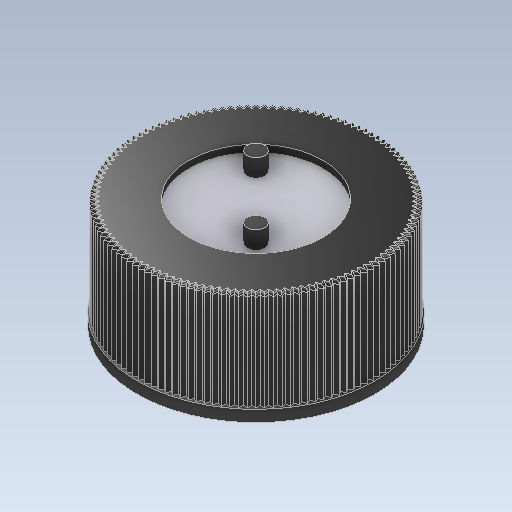
# Autodesk Inventor part: 40ml Bottle 1 lid
Saved by Autodesk Inventor 2021 (Build 250183000, 183)
## iProperties
Created: 2019-11-05
Part Number: 40ml Bottle 1 lid
Material: Generic
Document SubType Name: Modeling
Designer: jgray
Density: 1 g/cm^3
Appearance: Default
Author: jgray
Autodesk Inventor part; units mm, degrees
ref_plane "YZ Plane" through (0, 0, 0) normal (1, 0, 0) x (0, 1, 0)
ref_plane "XZ Plane" through (0, 0, 0) normal (0, 1, 0) x (-1, 0, 0)
ref_plane "XY Plane" through (0, 0, 0) normal (0, 0, 1) x (1, 0, 0)
sketch "Sketch1" plane through (0, 0, 0) normal (0, 1, 0) x (-1, 0, 0)
  circle A0 centre (0, 0) radius 13.35
  dimension "d0" = 26.7
  constraints: 1 centre point, 1 coincident
  measures "d0" diameter of A0
extrude "Extrusion1" add sketch "Sketch1" along normal blind 1.3
sketch "Sketch2" plane through (0, 1.3, 0) normal (0, 1, 0) x (1, 0, 0)
  circle A0 centre (0, 0) radius 13.2
  circle A1 centre (0, 0) radius 12.8 construction
  line L0 (-13.2, 0) -> (-13.1819, 0.6908) construction
  line L1 (-13.1819, 0.6908) -> (-13.1277, 1.3798) construction
  line L2 (-13.1277, 1.3798) -> (-13.0375, 2.0649) construction
  line L3 (-13.0375, 2.0649) -> (-12.9115, 2.7444) construction
  line L4 (-12.9115, 2.7444) -> (-12.7502, 3.4164) construction
  line L5 (-12.7502, 3.4164) -> (-12.5539, 4.079) construction
  line L6 (-12.5539, 4.079) -> (-12.3233, 4.7305) construction
  line L7 (-12.3233, 4.7305) -> (-12.0588, 5.3689) construction
  line L8 (-12.0588, 5.3689) -> (-11.7613, 5.9927) construction
  line L9 (-11.7613, 5.9927) -> (-11.4315, 6.6) construction
  line L10 (-11.4315, 6.6) -> (-11.0705, 7.1892) construction
  line L11 (-11.0705, 7.1892) -> (-10.679, 7.7588) construction
  line L12 (-10.679, 7.7588) -> (-10.2583, 8.307) construction
  line L13 (-10.2583, 8.307) -> (-9.8095, 8.8325) construction
  line L14 (-9.8095, 8.8325) -> (-9.3338, 9.3338) construction
  line L15 (-9.3338, 9.3338) -> (-8.8325, 9.8095) construction
  line L16 (-8.8325, 9.8095) -> (-8.307, 10.2583) construction
  line L17 (-8.307, 10.2583) -> (-7.7588, 10.679) construction
  line L18 (-7.7588, 10.679) -> (-7.1892, 11.0705) construction
  line L19 (-7.1892, 11.0705) -> (-6.6, 11.4315) construction
  line L20 (-6.6, 11.4315) -> (-5.9927, 11.7613) construction
  line L21 (-5.9927, 11.7613) -> (-5.3689, 12.0588) construction
  line L22 (-5.3689, 12.0588) -> (-4.7305, 12.3233) construction
  line L23 (-4.7305, 12.3233) -> (-4.079, 12.5539) construction
  line L24 (-4.079, 12.5539) -> (-3.4164, 12.7502) construction
  line L25 (-3.4164, 12.7502) -> (-2.7444, 12.9115) construction
  line L26 (-2.7444, 12.9115) -> (-2.0649, 13.0375) construction
  line L27 (-2.0649, 13.0375) -> (-1.3798, 13.1277) construction
  line L28 (-1.3798, 13.1277) -> (-0.6908, 13.1819) construction
  line L29 (-0.6908, 13.1819) -> (0, 13.2) construction
  line L30 (0, 13.2) -> (0.6908, 13.1819) construction
  line L31 (0.6908, 13.1819) -> (1.3798, 13.1277) construction
  line L32 (1.3798, 13.1277) -> (2.0649, 13.0375) construction
  line L33 (2.0649, 13.0375) -> (2.7444, 12.9115) construction
  line L34 (2.7444, 12.9115) -> (3.4164, 12.7502) construction
  line L35 (3.4164, 12.7502) -> (4.079, 12.5539) construction
  line L36 (4.079, 12.5539) -> (4.7305, 12.3233) construction
  line L37 (4.7305, 12.3233) -> (5.3689, 12.0588) construction
  line L38 (5.3689, 12.0588) -> (5.9927, 11.7613) construction
  line L39 (5.9927, 11.7613) -> (6.6, 11.4315) construction
  line L40 (6.6, 11.4315) -> (7.1892, 11.0705) construction
  line L41 (7.1892, 11.0705) -> (7.7588, 10.679) construction
  line L42 (7.7588, 10.679) -> (8.307, 10.2583) construction
  line L43 (8.307, 10.2583) -> (8.8325, 9.8095) construction
  line L44 (8.8325, 9.8095) -> (9.3338, 9.3338) construction
  line L45 (9.3338, 9.3338) -> (9.8095, 8.8325) construction
  line L46 (9.8095, 8.8325) -> (10.2583, 8.307) construction
  line L47 (10.2583, 8.307) -> (10.679, 7.7588) construction
  line L48 (10.679, 7.7588) -> (11.0705, 7.1892) construction
  line L49 (11.0705, 7.1892) -> (11.4315, 6.6) construction
  line L50 (11.4315, 6.6) -> (11.7613, 5.9927) construction
  line L51 (11.7613, 5.9927) -> (12.0588, 5.3689) construction
  line L52 (12.0588, 5.3689) -> (12.3233, 4.7305) construction
  line L53 (12.3233, 4.7305) -> (12.5539, 4.079) construction
  line L54 (12.5539, 4.079) -> (12.7502, 3.4164) construction
  line L55 (12.7502, 3.4164) -> (12.9115, 2.7444) construction
  line L56 (12.9115, 2.7444) -> (13.0375, 2.0649) construction
  line L57 (13.0375, 2.0649) -> (13.1277, 1.3798) construction
  line L58 (13.1277, 1.3798) -> (13.1819, 0.6908) construction
  line L59 (13.1819, 0.6908) -> (13.2, 0) construction
  line L60 (13.2, 0) -> (13.1819, -0.6908) construction
  line L61 (13.1819, -0.6908) -> (13.1277, -1.3798) construction
  line L62 (13.1277, -1.3798) -> (13.0375, -2.0649) construction
  line L63 (13.0375, -2.0649) -> (12.9115, -2.7444) construction
  line L64 (12.9115, -2.7444) -> (12.7502, -3.4164) construction
  line L65 (12.7502, -3.4164) -> (12.5539, -4.079) construction
  line L66 (12.5539, -4.079) -> (12.3233, -4.7305) construction
  line L67 (12.3233, -4.7305) -> (12.0588, -5.3689) construction
  line L68 (12.0588, -5.3689) -> (11.7613, -5.9927) construction
  line L69 (11.7613, -5.9927) -> (11.4315, -6.6) construction
  line L70 (11.4315, -6.6) -> (11.0705, -7.1892) construction
  line L71 (11.0705, -7.1892) -> (10.679, -7.7588) construction
  line L72 (10.679, -7.7588) -> (10.2583, -8.307) construction
  line L73 (10.2583, -8.307) -> (9.8095, -8.8325) construction
  line L74 (9.8095, -8.8325) -> (9.3338, -9.3338) construction
  line L75 (9.3338, -9.3338) -> (8.8325, -9.8095) construction
  line L76 (8.8325, -9.8095) -> (8.307, -10.2583) construction
  line L77 (8.307, -10.2583) -> (7.7588, -10.679) construction
  line L78 (7.7588, -10.679) -> (7.1892, -11.0705) construction
  line L79 (7.1892, -11.0705) -> (6.6, -11.4315) construction
  line L80 (6.6, -11.4315) -> (5.9927, -11.7613) construction
  line L81 (5.9927, -11.7613) -> (5.3689, -12.0588) construction
  line L82 (5.3689, -12.0588) -> (4.7305, -12.3233) construction
  line L83 (4.7305, -12.3233) -> (4.079, -12.5539) construction
  line L84 (4.079, -12.5539) -> (3.4164, -12.7502) construction
  line L85 (3.4164, -12.7502) -> (2.7444, -12.9115) construction
  line L86 (2.7444, -12.9115) -> (2.0649, -13.0375) construction
  line L87 (2.0649, -13.0375) -> (1.3798, -13.1277) construction
  line L88 (1.3798, -13.1277) -> (0.6908, -13.1819) construction
  line L89 (0.6908, -13.1819) -> (0, -13.2) construction
  line L90 (0, -13.2) -> (-0.6908, -13.1819) construction
  line L91 (-0.6908, -13.1819) -> (-1.3798, -13.1277) construction
  line L92 (-1.3798, -13.1277) -> (-2.0649, -13.0375) construction
  line L93 (-2.0649, -13.0375) -> (-2.7444, -12.9115) construction
  line L94 (-2.7444, -12.9115) -> (-3.4164, -12.7502) construction
  line L95 (-3.4164, -12.7502) -> (-4.079, -12.5539) construction
  line L96 (-4.079, -12.5539) -> (-4.7305, -12.3233) construction
  line L97 (-4.7305, -12.3233) -> (-5.3689, -12.0588) construction
  line L98 (-5.3689, -12.0588) -> (-5.9927, -11.7613) construction
  line L99 (-5.9927, -11.7613) -> (-6.6, -11.4315) construction
  line L100 (-6.6, -11.4315) -> (-7.1892, -11.0705) construction
  line L101 (-7.1892, -11.0705) -> (-7.7588, -10.679) construction
  line L102 (-7.7588, -10.679) -> (-8.307, -10.2583) construction
  line L103 (-8.307, -10.2583) -> (-8.8325, -9.8095) construction
  line L104 (-8.8325, -9.8095) -> (-9.3338, -9.3338) construction
  line L105 (-9.3338, -9.3338) -> (-9.8095, -8.8325) construction
  line L106 (-9.8095, -8.8325) -> (-10.2583, -8.307) construction
  line L107 (-10.2583, -8.307) -> (-10.679, -7.7588) construction
  line L108 (-10.679, -7.7588) -> (-11.0705, -7.1892) construction
  line L109 (-11.0705, -7.1892) -> (-11.4315, -6.6) construction
  line L110 (-11.4315, -6.6) -> (-11.7613, -5.9927) construction
  line L111 (-11.7613, -5.9927) -> (-12.0588, -5.3689) construction
  line L112 (-12.0588, -5.3689) -> (-12.3233, -4.7305) construction
  line L113 (-12.3233, -4.7305) -> (-12.5539, -4.079) construction
  line L114 (-12.5539, -4.079) -> (-12.7502, -3.4164) construction
  line L115 (-12.7502, -3.4164) -> (-12.9115, -2.7444) construction
  line L116 (-12.9115, -2.7444) -> (-13.0375, -2.0649) construction
  line L117 (-13.0375, -2.0649) -> (-13.1277, -1.3798) construction
  line L118 (-13.1277, -1.3798) -> (-13.1819, -0.6908) construction
  line L119 (-13.1819, -0.6908) -> (-13.2, 0) construction
  line L120 (0, 0) -> (-13.191, -0.3454) construction
  line L121 (-12.7956, -0.3351) -> (-12.7956, 0.3351) construction
  line L122 (-12.7956, 0.3351) -> (-12.7605, 1.0043) construction
  line L123 (-12.7605, 1.0043) -> (-12.6905, 1.6707) construction
  line L124 (-12.6905, 1.6707) -> (-12.5857, 2.3326) construction
  line L125 (-12.5857, 2.3326) -> (-12.4463, 2.9881) construction
  line L126 (-12.4463, 2.9881) -> (-12.2729, 3.6354) construction
  line L127 (-12.2729, 3.6354) -> (-12.0658, 4.2727) construction
  line L128 (-12.0658, 4.2727) -> (-11.8257, 4.8983) construction
  line L129 (-11.8257, 4.8983) -> (-11.5531, 5.5105) construction
  line L130 (-11.5531, 5.5105) -> (-11.2489, 6.1076) construction
  line L131 (-11.2489, 6.1076) -> (-10.9138, 6.688) construction
  line L132 (-10.9138, 6.688) -> (-10.5488, 7.25) construction
  line L133 (-10.5488, 7.25) -> (-10.1549, 7.7921) construction
  line L134 (-10.1549, 7.7921) -> (-9.7332, 8.3129) construction
  line L135 (-9.7332, 8.3129) -> (-9.2848, 8.8109) construction
  line L136 (-9.2848, 8.8109) -> (-8.8109, 9.2848) construction
  line L137 (-8.8109, 9.2848) -> (-8.3129, 9.7332) construction
  line L138 (-8.3129, 9.7332) -> (-7.7921, 10.1549) construction
  line L139 (-7.7921, 10.1549) -> (-7.25, 10.5488) construction
  line L140 (-7.25, 10.5488) -> (-6.688, 10.9138) construction
  line L141 (-6.688, 10.9138) -> (-6.1076, 11.2489) construction
  line L142 (-6.1076, 11.2489) -> (-5.5105, 11.5531) construction
  line L143 (-5.5105, 11.5531) -> (-4.8983, 11.8257) construction
  line L144 (-4.8983, 11.8257) -> (-4.2727, 12.0658) construction
  line L145 (-4.2727, 12.0658) -> (-3.6354, 12.2729) construction
  line L146 (-3.6354, 12.2729) -> (-2.9881, 12.4463) construction
  line L147 (-2.9881, 12.4463) -> (-2.3326, 12.5857) construction
  line L148 (-2.3326, 12.5857) -> (-1.6707, 12.6905) construction
  line L149 (-1.6707, 12.6905) -> (-1.0043, 12.7605) construction
  line L150 (-1.0043, 12.7605) -> (-0.3351, 12.7956) construction
  line L151 (-0.3351, 12.7956) -> (0.3351, 12.7956) construction
  line L152 (0.3351, 12.7956) -> (1.0043, 12.7605) construction
  line L153 (1.0043, 12.7605) -> (1.6707, 12.6905) construction
  line L154 (1.6707, 12.6905) -> (2.3326, 12.5857) construction
  line L155 (2.3326, 12.5857) -> (2.9881, 12.4463) construction
  line L156 (2.9881, 12.4463) -> (3.6354, 12.2729) construction
  line L157 (3.6354, 12.2729) -> (4.2727, 12.0658) construction
  line L158 (4.2727, 12.0658) -> (4.8983, 11.8257) construction
  line L159 (4.8983, 11.8257) -> (5.5105, 11.5531) construction
  line L160 (5.5105, 11.5531) -> (6.1076, 11.2489) construction
  line L161 (6.1076, 11.2489) -> (6.688, 10.9138) construction
  line L162 (6.688, 10.9138) -> (7.25, 10.5488) construction
  line L163 (7.25, 10.5488) -> (7.7921, 10.1549) construction
  line L164 (7.7921, 10.1549) -> (8.3129, 9.7332) construction
  line L165 (8.3129, 9.7332) -> (8.8109, 9.2848) construction
  line L166 (8.8109, 9.2848) -> (9.2848, 8.8109) construction
  line L167 (9.2848, 8.8109) -> (9.7332, 8.3129) construction
  line L168 (9.7332, 8.3129) -> (10.1549, 7.7921) construction
  line L169 (10.1549, 7.7921) -> (10.5488, 7.25) construction
  line L170 (10.5488, 7.25) -> (10.9138, 6.688) construction
  line L171 (10.9138, 6.688) -> (11.2489, 6.1076) construction
  line L172 (11.2489, 6.1076) -> (11.5531, 5.5105) construction
  line L173 (11.5531, 5.5105) -> (11.8257, 4.8983) construction
  line L174 (11.8257, 4.8983) -> (12.0658, 4.2727) construction
  line L175 (12.0658, 4.2727) -> (12.2729, 3.6354) construction
  line L176 (12.2729, 3.6354) -> (12.4463, 2.9881) construction
  line L177 (12.4463, 2.9881) -> (12.5857, 2.3326) construction
  line L178 (12.5857, 2.3326) -> (12.6905, 1.6707) construction
  line L179 (12.6905, 1.6707) -> (12.7605, 1.0043) construction
  line L180 (12.7605, 1.0043) -> (12.7956, 0.3351) construction
  line L181 (12.7956, 0.3351) -> (12.7956, -0.3351) construction
  line L182 (12.7956, -0.3351) -> (12.7605, -1.0043) construction
  line L183 (12.7605, -1.0043) -> (12.6905, -1.6707) construction
  line L184 (12.6905, -1.6707) -> (12.5857, -2.3326) construction
  line L185 (12.5857, -2.3326) -> (12.4463, -2.9881) construction
  line L186 (12.4463, -2.9881) -> (12.2729, -3.6354) construction
  line L187 (12.2729, -3.6354) -> (12.0658, -4.2727) construction
  line L188 (12.0658, -4.2727) -> (11.8257, -4.8983) construction
  line L189 (11.8257, -4.8983) -> (11.5531, -5.5105) construction
  line L190 (11.5531, -5.5105) -> (11.2489, -6.1076) construction
  line L191 (11.2489, -6.1076) -> (10.9138, -6.688) construction
  line L192 (10.9138, -6.688) -> (10.5488, -7.25) construction
  line L193 (10.5488, -7.25) -> (10.1549, -7.7921) construction
  line L194 (10.1549, -7.7921) -> (9.7332, -8.3129) construction
  line L195 (9.7332, -8.3129) -> (9.2848, -8.8109) construction
  line L196 (9.2848, -8.8109) -> (8.8109, -9.2848) construction
  line L197 (8.8109, -9.2848) -> (8.3129, -9.7332) construction
  line L198 (8.3129, -9.7332) -> (7.7921, -10.1549) construction
  line L199 (7.7921, -10.1549) -> (7.25, -10.5488) construction
  line L200 (7.25, -10.5488) -> (6.688, -10.9138) construction
  line L201 (6.688, -10.9138) -> (6.1076, -11.2489) construction
  line L202 (6.1076, -11.2489) -> (5.5105, -11.5531) construction
  line L203 (5.5105, -11.5531) -> (4.8983, -11.8257) construction
  line L204 (4.8983, -11.8257) -> (4.2727, -12.0658) construction
  line L205 (4.2727, -12.0658) -> (3.6354, -12.2729) construction
  line L206 (3.6354, -12.2729) -> (2.9881, -12.4463) construction
  line L207 (2.9881, -12.4463) -> (2.3326, -12.5857) construction
  line L208 (2.3326, -12.5857) -> (1.6707, -12.6905) construction
  line L209 (1.6707, -12.6905) -> (1.0043, -12.7605) construction
  line L210 (1.0043, -12.7605) -> (0.3351, -12.7956) construction
  line L211 (0.3351, -12.7956) -> (-0.3351, -12.7956) construction
  line L212 (-0.3351, -12.7956) -> (-1.0043, -12.7605) construction
  line L213 (-1.0043, -12.7605) -> (-1.6707, -12.6905) construction
  line L214 (-1.6707, -12.6905) -> (-2.3326, -12.5857) construction
  line L215 (-2.3326, -12.5857) -> (-2.9881, -12.4463) construction
  line L216 (-2.9881, -12.4463) -> (-3.6354, -12.2729) construction
  line L217 (-3.6354, -12.2729) -> (-4.2727, -12.0658) construction
  line L218 (-4.2727, -12.0658) -> (-4.8983, -11.8257) construction
  line L219 (-4.8983, -11.8257) -> (-5.5105, -11.5531) construction
  line L220 (-5.5105, -11.5531) -> (-6.1076, -11.2489) construction
  line L221 (-6.1076, -11.2489) -> (-6.688, -10.9138) construction
  line L222 (-6.688, -10.9138) -> (-7.25, -10.5488) construction
  line L223 (-7.25, -10.5488) -> (-7.7921, -10.1549) construction
  line L224 (-7.7921, -10.1549) -> (-8.3129, -9.7332) construction
  line L225 (-8.3129, -9.7332) -> (-8.8109, -9.2848) construction
  line L226 (-8.8109, -9.2848) -> (-9.2848, -8.8109) construction
  line L227 (-9.2848, -8.8109) -> (-9.7332, -8.3129) construction
  line L228 (-9.7332, -8.3129) -> (-10.1549, -7.7921) construction
  line L229 (-10.1549, -7.7921) -> (-10.5488, -7.25) construction
  line L230 (-10.5488, -7.25) -> (-10.9138, -6.688) construction
  line L231 (-10.9138, -6.688) -> (-11.2489, -6.1076) construction
  line L232 (-11.2489, -6.1076) -> (-11.5531, -5.5105) construction
  line L233 (-11.5531, -5.5105) -> (-11.8257, -4.8983) construction
  line L234 (-11.8257, -4.8983) -> (-12.0658, -4.2727) construction
  line L235 (-12.0658, -4.2727) -> (-12.2729, -3.6354) construction
  line L236 (-12.2729, -3.6354) -> (-12.4463, -2.9881) construction
  line L237 (-12.4463, -2.9881) -> (-12.5857, -2.3326) construction
  line L238 (-12.5857, -2.3326) -> (-12.6905, -1.6707) construction
  line L239 (-12.6905, -1.6707) -> (-12.7605, -1.0043) construction
  line L240 (-12.7605, -1.0043) -> (-12.7956, -0.3351) construction
  line L241 (-12.7956, -0.3351) -> (-13.2, 0)
  line L242 (-12.7956, 0.3351) -> (-13.2, 0)
  line L243 (-12.7605, -1.0043) -> (-13.1819, -0.6908)
  line L244 (-12.7956, -0.3351) -> (-13.1819, -0.6908)
  line L245 (-12.6905, -1.6707) -> (-13.1277, -1.3798)
  line L246 (-12.7605, -1.0043) -> (-13.1277, -1.3798)
  line L247 (-12.5857, -2.3326) -> (-13.0375, -2.0649)
  line L248 (-12.6905, -1.6707) -> (-13.0375, -2.0649)
  line L249 (-12.4463, -2.9881) -> (-12.9115, -2.7444)
  line L250 (-12.5857, -2.3326) -> (-12.9115, -2.7444)
  line L251 (-12.2729, -3.6354) -> (-12.7502, -3.4164)
  line L252 (-12.4463, -2.9881) -> (-12.7502, -3.4164)
  line L253 (-12.0658, -4.2727) -> (-12.5539, -4.079)
  line L254 (-12.2729, -3.6354) -> (-12.5539, -4.079)
  line L255 (-11.8257, -4.8983) -> (-12.3233, -4.7305)
  line L256 (-12.0658, -4.2727) -> (-12.3233, -4.7305)
  line L257 (-11.5531, -5.5105) -> (-12.0588, -5.3689)
  line L258 (-11.8257, -4.8983) -> (-12.0588, -5.3689)
  line L259 (-11.2489, -6.1076) -> (-11.7613, -5.9927)
  line L260 (-11.5531, -5.5105) -> (-11.7613, -5.9927)
  line L261 (-10.9138, -6.688) -> (-11.4315, -6.6)
  line L262 (-11.2489, -6.1076) -> (-11.4315, -6.6)
  line L263 (-10.5488, -7.25) -> (-11.0705, -7.1892)
  line L264 (-10.9138, -6.688) -> (-11.0705, -7.1892)
  line L265 (-10.1549, -7.7921) -> (-10.679, -7.7588)
  line L266 (-10.5488, -7.25) -> (-10.679, -7.7588)
  line L267 (-9.7332, -8.3129) -> (-10.2583, -8.307)
  line L268 (-10.1549, -7.7921) -> (-10.2583, -8.307)
  line L269 (-9.2848, -8.8109) -> (-9.8095, -8.8325)
  line L270 (-9.7332, -8.3129) -> (-9.8095, -8.8325)
  line L271 (-8.8109, -9.2848) -> (-9.3338, -9.3338)
  line L272 (-9.2848, -8.8109) -> (-9.3338, -9.3338)
  line L273 (-8.3129, -9.7332) -> (-8.8325, -9.8095)
  line L274 (-8.8109, -9.2848) -> (-8.8325, -9.8095)
  line L275 (-7.7921, -10.1549) -> (-8.307, -10.2583)
  line L276 (-8.3129, -9.7332) -> (-8.307, -10.2583)
  line L277 (-7.25, -10.5488) -> (-7.7588, -10.679)
  line L278 (-7.7921, -10.1549) -> (-7.7588, -10.679)
  line L279 (-6.688, -10.9138) -> (-7.1892, -11.0705)
  line L280 (-7.25, -10.5488) -> (-7.1892, -11.0705)
  line L281 (-6.1076, -11.2489) -> (-6.6, -11.4315)
  line L282 (-6.688, -10.9138) -> (-6.6, -11.4315)
  line L283 (-5.5105, -11.5531) -> (-5.9927, -11.7613)
  line L284 (-6.1076, -11.2489) -> (-5.9927, -11.7613)
  line L285 (-4.8983, -11.8257) -> (-5.3689, -12.0588)
  line L286 (-5.5105, -11.5531) -> (-5.3689, -12.0588)
  line L287 (-4.2727, -12.0658) -> (-4.7305, -12.3233)
  line L288 (-4.8983, -11.8257) -> (-4.7305, -12.3233)
  line L289 (-3.6354, -12.2729) -> (-4.079, -12.5539)
  line L290 (-4.2727, -12.0658) -> (-4.079, -12.5539)
  line L291 (-2.9881, -12.4463) -> (-3.4164, -12.7502)
  line L292 (-3.6354, -12.2729) -> (-3.4164, -12.7502)
  line L293 (-2.3326, -12.5857) -> (-2.7444, -12.9115)
  line L294 (-2.9881, -12.4463) -> (-2.7444, -12.9115)
  line L295 (-1.6707, -12.6905) -> (-2.0649, -13.0375)
  line L296 (-2.3326, -12.5857) -> (-2.0649, -13.0375)
  line L297 (-1.0043, -12.7605) -> (-1.3798, -13.1277)
  line L298 (-1.6707, -12.6905) -> (-1.3798, -13.1277)
  line L299 (-0.3351, -12.7956) -> (-0.6908, -13.1819)
  line L300 (-1.0043, -12.7605) -> (-0.6908, -13.1819)
  line L301 (0.3351, -12.7956) -> (0, -13.2)
  line L302 (-0.3351, -12.7956) -> (0, -13.2)
  line L303 (1.0043, -12.7605) -> (0.6908, -13.1819)
  line L304 (0.3351, -12.7956) -> (0.6908, -13.1819)
  line L305 (1.6707, -12.6905) -> (1.3798, -13.1277)
  line L306 (1.0043, -12.7605) -> (1.3798, -13.1277)
  line L307 (2.3326, -12.5857) -> (2.0649, -13.0375)
  line L308 (1.6707, -12.6905) -> (2.0649, -13.0375)
  line L309 (2.9881, -12.4463) -> (2.7444, -12.9115)
  line L310 (2.3326, -12.5857) -> (2.7444, -12.9115)
  line L311 (3.6354, -12.2729) -> (3.4164, -12.7502)
  line L312 (2.9881, -12.4463) -> (3.4164, -12.7502)
  line L313 (4.2727, -12.0658) -> (4.079, -12.5539)
  line L314 (3.6354, -12.2729) -> (4.079, -12.5539)
  line L315 (4.8983, -11.8257) -> (4.7305, -12.3233)
  line L316 (4.2727, -12.0658) -> (4.7305, -12.3233)
  line L317 (5.5105, -11.5531) -> (5.3689, -12.0588)
  line L318 (4.8983, -11.8257) -> (5.3689, -12.0588)
  line L319 (6.1076, -11.2489) -> (5.9927, -11.7613)
  line L320 (5.5105, -11.5531) -> (5.9927, -11.7613)
  line L321 (6.688, -10.9138) -> (6.6, -11.4315)
  line L322 (6.1076, -11.2489) -> (6.6, -11.4315)
  line L323 (7.25, -10.5488) -> (7.1892, -11.0705)
  line L324 (6.688, -10.9138) -> (7.1892, -11.0705)
  line L325 (7.7921, -10.1549) -> (7.7588, -10.679)
  line L326 (7.25, -10.5488) -> (7.7588, -10.679)
  line L327 (8.3129, -9.7332) -> (8.307, -10.2583)
  line L328 (7.7921, -10.1549) -> (8.307, -10.2583)
  line L329 (8.8109, -9.2848) -> (8.8325, -9.8095)
  line L330 (8.3129, -9.7332) -> (8.8325, -9.8095)
  line L331 (9.2848, -8.8109) -> (9.3338, -9.3338)
  line L332 (8.8109, -9.2848) -> (9.3338, -9.3338)
  line L333 (9.7332, -8.3129) -> (9.8095, -8.8325)
  line L334 (9.2848, -8.8109) -> (9.8095, -8.8325)
  line L335 (10.1549, -7.7921) -> (10.2583, -8.307)
  line L336 (9.7332, -8.3129) -> (10.2583, -8.307)
  line L337 (10.5488, -7.25) -> (10.679, -7.7588)
  line L338 (10.1549, -7.7921) -> (10.679, -7.7588)
  line L339 (10.9138, -6.688) -> (11.0705, -7.1892)
  line L340 (10.5488, -7.25) -> (11.0705, -7.1892)
  line L341 (11.2489, -6.1076) -> (11.4315, -6.6)
  line L342 (10.9138, -6.688) -> (11.4315, -6.6)
  line L343 (11.5531, -5.5105) -> (11.7613, -5.9927)
  line L344 (11.2489, -6.1076) -> (11.7613, -5.9927)
  line L345 (11.8257, -4.8983) -> (12.0588, -5.3689)
  line L346 (11.5531, -5.5105) -> (12.0588, -5.3689)
  line L347 (12.0658, -4.2727) -> (12.3233, -4.7305)
  line L348 (11.8257, -4.8983) -> (12.3233, -4.7305)
  line L349 (12.2729, -3.6354) -> (12.5539, -4.079)
  line L350 (12.0658, -4.2727) -> (12.5539, -4.079)
  line L351 (12.4463, -2.9881) -> (12.7502, -3.4164)
  line L352 (12.2729, -3.6354) -> (12.7502, -3.4164)
  line L353 (12.5857, -2.3326) -> (12.9115, -2.7444)
  line L354 (12.4463, -2.9881) -> (12.9115, -2.7444)
  line L355 (12.6905, -1.6707) -> (13.0375, -2.0649)
  line L356 (12.5857, -2.3326) -> (13.0375, -2.0649)
  line L357 (12.7605, -1.0043) -> (13.1277, -1.3798)
  line L358 (12.6905, -1.6707) -> (13.1277, -1.3798)
  line L359 (12.7956, -0.3351) -> (13.1819, -0.6908)
  line L360 (12.7605, -1.0043) -> (13.1819, -0.6908)
  line L361 (12.7956, 0.3351) -> (13.2, 0)
  line L362 (12.7956, -0.3351) -> (13.2, 0)
  line L363 (12.7605, 1.0043) -> (13.1819, 0.6908)
  line L364 (12.7956, 0.3351) -> (13.1819, 0.6908)
  line L365 (12.6905, 1.6707) -> (13.1277, 1.3798)
  line L366 (12.7605, 1.0043) -> (13.1277, 1.3798)
  line L367 (12.5857, 2.3326) -> (13.0375, 2.0649)
  line L368 (12.6905, 1.6707) -> (13.0375, 2.0649)
  line L369 (12.4463, 2.9881) -> (12.9115, 2.7444)
  line L370 (12.5857, 2.3326) -> (12.9115, 2.7444)
  line L371 (12.2729, 3.6354) -> (12.7502, 3.4164)
  line L372 (12.4463, 2.9881) -> (12.7502, 3.4164)
  line L373 (12.0658, 4.2727) -> (12.5539, 4.079)
  line L374 (12.2729, 3.6354) -> (12.5539, 4.079)
  line L375 (11.8257, 4.8983) -> (12.3233, 4.7305)
  line L376 (12.0658, 4.2727) -> (12.3233, 4.7305)
  line L377 (11.5531, 5.5105) -> (12.0588, 5.3689)
  line L378 (11.8257, 4.8983) -> (12.0588, 5.3689)
  line L379 (11.2489, 6.1076) -> (11.7613, 5.9927)
  line L380 (11.5531, 5.5105) -> (11.7613, 5.9927)
  line L381 (10.9138, 6.688) -> (11.4315, 6.6)
  line L382 (11.2489, 6.1076) -> (11.4315, 6.6)
  line L383 (10.5488, 7.25) -> (11.0705, 7.1892)
  line L384 (10.9138, 6.688) -> (11.0705, 7.1892)
  line L385 (10.1549, 7.7921) -> (10.679, 7.7588)
  line L386 (10.5488, 7.25) -> (10.679, 7.7588)
  line L387 (9.7332, 8.3129) -> (10.2583, 8.307)
  line L388 (10.1549, 7.7921) -> (10.2583, 8.307)
  line L389 (9.2848, 8.8109) -> (9.8095, 8.8325)
  line L390 (9.7332, 8.3129) -> (9.8095, 8.8325)
  line L391 (8.8109, 9.2848) -> (9.3338, 9.3338)
  line L392 (9.2848, 8.8109) -> (9.3338, 9.3338)
  line L393 (8.3129, 9.7332) -> (8.8325, 9.8095)
  line L394 (8.8109, 9.2848) -> (8.8325, 9.8095)
  line L395 (7.7921, 10.1549) -> (8.307, 10.2583)
  line L396 (8.3129, 9.7332) -> (8.307, 10.2583)
  line L397 (7.25, 10.5488) -> (7.7588, 10.679)
  line L398 (7.7921, 10.1549) -> (7.7588, 10.679)
  line L399 (6.688, 10.9138) -> (7.1892, 11.0705)
  line L400 (7.25, 10.5488) -> (7.1892, 11.0705)
  line L401 (6.1076, 11.2489) -> (6.6, 11.4315)
  line L402 (6.688, 10.9138) -> (6.6, 11.4315)
  line L403 (5.5105, 11.5531) -> (5.9927, 11.7613)
  line L404 (6.1076, 11.2489) -> (5.9927, 11.7613)
  line L405 (4.8983, 11.8257) -> (5.3689, 12.0588)
  line L406 (5.5105, 11.5531) -> (5.3689, 12.0588)
  line L407 (4.2727, 12.0658) -> (4.7305, 12.3233)
  line L408 (4.8983, 11.8257) -> (4.7305, 12.3233)
  line L409 (3.6354, 12.2729) -> (4.079, 12.5539)
  line L410 (4.2727, 12.0658) -> (4.079, 12.5539)
  line L411 (2.9881, 12.4463) -> (3.4164, 12.7502)
  line L412 (3.6354, 12.2729) -> (3.4164, 12.7502)
  line L413 (2.3326, 12.5857) -> (2.7444, 12.9115)
  line L414 (2.9881, 12.4463) -> (2.7444, 12.9115)
  line L415 (1.6707, 12.6905) -> (2.0649, 13.0375)
  line L416 (2.3326, 12.5857) -> (2.0649, 13.0375)
  line L417 (1.0043, 12.7605) -> (1.3798, 13.1277)
  line L418 (1.6707, 12.6905) -> (1.3798, 13.1277)
  line L419 (0.3351, 12.7956) -> (0.6908, 13.1819)
  line L420 (1.0043, 12.7605) -> (0.6908, 13.1819)
  line L421 (-0.3351, 12.7956) -> (0, 13.2)
  line L422 (0.3351, 12.7956) -> (0, 13.2)
  line L423 (-1.0043, 12.7605) -> (-0.6908, 13.1819)
  line L424 (-0.3351, 12.7956) -> (-0.6908, 13.1819)
  line L425 (-1.6707, 12.6905) -> (-1.3798, 13.1277)
  line L426 (-1.0043, 12.7605) -> (-1.3798, 13.1277)
  line L427 (-2.3326, 12.5857) -> (-2.0649, 13.0375)
  line L428 (-1.6707, 12.6905) -> (-2.0649, 13.0375)
  line L429 (-2.9881, 12.4463) -> (-2.7444, 12.9115)
  line L430 (-2.3326, 12.5857) -> (-2.7444, 12.9115)
  line L431 (-3.6354, 12.2729) -> (-3.4164, 12.7502)
  line L432 (-2.9881, 12.4463) -> (-3.4164, 12.7502)
  line L433 (-4.2727, 12.0658) -> (-4.079, 12.5539)
  line L434 (-3.6354, 12.2729) -> (-4.079, 12.5539)
  line L435 (-4.8983, 11.8257) -> (-4.7305, 12.3233)
  line L436 (-4.2727, 12.0658) -> (-4.7305, 12.3233)
  line L437 (-5.5105, 11.5531) -> (-5.3689, 12.0588)
  line L438 (-4.8983, 11.8257) -> (-5.3689, 12.0588)
  line L439 (-6.1076, 11.2489) -> (-5.9927, 11.7613)
  line L440 (-5.5105, 11.5531) -> (-5.9927, 11.7613)
  line L441 (-6.688, 10.9138) -> (-6.6, 11.4315)
  line L442 (-6.1076, 11.2489) -> (-6.6, 11.4315)
  line L443 (-7.25, 10.5488) -> (-7.1892, 11.0705)
  line L444 (-6.688, 10.9138) -> (-7.1892, 11.0705)
  line L445 (-7.7921, 10.1549) -> (-7.7588, 10.679)
  line L446 (-7.25, 10.5488) -> (-7.7588, 10.679)
  line L447 (-8.3129, 9.7332) -> (-8.307, 10.2583)
  line L448 (-7.7921, 10.1549) -> (-8.307, 10.2583)
  line L449 (-8.8109, 9.2848) -> (-8.8325, 9.8095)
  line L450 (-8.3129, 9.7332) -> (-8.8325, 9.8095)
  line L451 (-9.2848, 8.8109) -> (-9.3338, 9.3338)
  line L452 (-8.8109, 9.2848) -> (-9.3338, 9.3338)
  line L453 (-9.7332, 8.3129) -> (-9.8095, 8.8325)
  line L454 (-9.2848, 8.8109) -> (-9.8095, 8.8325)
  line L455 (-10.1549, 7.7921) -> (-10.2583, 8.307)
  line L456 (-9.7332, 8.3129) -> (-10.2583, 8.307)
  line L457 (-10.5488, 7.25) -> (-10.679, 7.7588)
  line L458 (-10.1549, 7.7921) -> (-10.679, 7.7588)
  line L459 (-10.9138, 6.688) -> (-11.0705, 7.1892)
  line L460 (-10.5488, 7.25) -> (-11.0705, 7.1892)
  line L461 (-11.2489, 6.1076) -> (-11.4315, 6.6)
  line L462 (-10.9138, 6.688) -> (-11.4315, 6.6)
  line L463 (-11.5531, 5.5105) -> (-11.7613, 5.9927)
  line L464 (-11.2489, 6.1076) -> (-11.7613, 5.9927)
  line L465 (-11.8257, 4.8983) -> (-12.0588, 5.3689)
  line L466 (-11.5531, 5.5105) -> (-12.0588, 5.3689)
  line L467 (-12.0658, 4.2727) -> (-12.3233, 4.7305)
  line L468 (-11.8257, 4.8983) -> (-12.3233, 4.7305)
  line L469 (-12.2729, 3.6354) -> (-12.5539, 4.079)
  line L470 (-12.0658, 4.2727) -> (-12.5539, 4.079)
  line L471 (-12.4463, 2.9881) -> (-12.7502, 3.4164)
  line L472 (-12.2729, 3.6354) -> (-12.7502, 3.4164)
  line L473 (-12.5857, 2.3326) -> (-12.9115, 2.7444)
  line L474 (-12.4463, 2.9881) -> (-12.9115, 2.7444)
  line L475 (-12.6905, 1.6707) -> (-13.0375, 2.0649)
  line L476 (-12.5857, 2.3326) -> (-13.0375, 2.0649)
  line L477 (-12.7605, 1.0043) -> (-13.1277, 1.3798)
  line L478 (-12.6905, 1.6707) -> (-13.1277, 1.3798)
  line L479 (-12.7956, 0.3351) -> (-13.1819, 0.6908)
  line L480 (-12.7605, 1.0043) -> (-13.1819, 0.6908)
  dimension "d7" = 360
  constraints: 962 end point, 4 coincident, 1 horizontal alignment, 1 midpoint, 1 point on line, 1088 other
extrude "Extrusion2" add sketch "Sketch2" along normal blind 11 contours L362 L359 L360 L357 L358 L355 L356 L353 L354 L351 L352 L349 L350 L347 L348 L345 L346 L343 L344 L341 L342 L339 L340 L337 L338 L335 L336 L333 L334 L331 L332 L329 L330 L327 L328 L325 L326 L323 L324 L321 L322 L319 L320 L317 L318 L315 L316 L313 L314 L311 L312 L309 L310 L307 L308 L305 L306 L303 L304 L301 L302 L299 L300 L297 L298 L295 L296 L293 L294 L291 L292 L289 L290 L287 L288 L285 L286 L283 L284 L281 L282 L279 L280 L277 L278 L275 L276 L273 L274 L271 L272 L269 L270 L267 L268 L265 L266 L263 L264 L261 L262 L259 L260 L257 L258 L255 L256 L253 L254 L251 L252 L249 L250 L247 L248 L245 L246 L243 L244 L241 L242 L479 L480 L477 L478 L475 L476 L473 L474 L471 L472 L469 L470 L467 L468 L465 L466 L463 L464 L461 L462 L459 L460 L457 L458 L455 L456 L453 L454 L451 L452 L449 L450 L447 L448 L445 L446 L443 L444 L441 L442 L439 L440 L437 L438 L435 L436 L433 L434 L431 L432 L429 L430 L427 L428 L425 L426 L423 L424 L421 L422 L419 L420 L417 L418 L415 L416 L413 L414 L411 L412 L409 L410 L407 L408 L405 L406 L403 L404 L401 L402 L399 L400 L397 L398 L395 L396 L393 L394 L391 L392 L389 L390 L387 L388 L385 L386 L383 L384 L381 L382 L379 L380 L377 L378 L375 L376 L373 L374 L371 L372 L369 L370 L367 L368 L365 L366 L363 L364 L361
sketch "Sketch3" plane through (0, 12.3, 0) normal (0, 1, 0) x (1, 0, 0)
  line L0 (-13.2, 0) -> (-12.7956, -0.3351) projected
  circle A0 centre (0, 0) radius 13.2
  constraints: 1 coincident, 1 horizontal alignment, 2 other
fillet "Fillet1" radius 0.25 240 edges at (-10.8096, 12.3, -7.2196) (-10.9921, 12.3, -6.9386) (-11.1727, 12.3, -6.644) (-11.3402, 12.3, -6.3538) (-11.5051, 12.3, -6.0502) (-11.6572, 12.3, -5.7516) (-11.8059, 12.3, -5.4397) (-11.9422, 12.3, -5.1336) (-12.0745, 12.3, -4.8144) (-12.1945, 12.3, -4.5016) (-12.3099, 12.3, -4.1759) (-12.4134, 12.3, -3.8572) (-12.5116, 12.3, -3.5259) (-12.5983, 12.3, -3.2023) (-12.6789, 12.3, -2.8663) (-12.7486, 12.3, -2.5385) (-12.8116, 12.3, -2.1988) (-12.864, 12.3, -1.8678) (-12.9091, 12.3, -1.5253) (-12.9441, 12.3, -1.192) (-12.9712, 12.3, -0.8476) (-12.9888, 12.3, -0.5129) (-12.9978, 12.3, -0.1675) (-12.9978, 12.3, 0.1675) (-12.9888, 12.3, 0.5129) (-12.9712, 12.3, 0.8476) (-12.9441, 12.3, 1.192) (-12.9091, 12.3, 1.5253) (-12.864, 12.3, 1.8678) (-12.8116, 12.3, 2.1988) (-12.7486, 12.3, 2.5385) (-12.6789, 12.3, 2.8663) (-12.5983, 12.3, 3.2023) (-12.5116, 12.3, 3.5259) (-12.4134, 12.3, 3.8572) (-12.3099, 12.3, 4.1759) (-12.1945, 12.3, 4.5016) (-12.0745, 12.3, 4.8144) (-11.9422, 12.3, 5.1336) (-11.8059, 12.3, 5.4397) (-11.6572, 12.3, 5.7516) (-11.5051, 12.3, 6.0502) (-11.3402, 12.3, 6.3538) (-11.1727, 12.3, 6.644) (-10.9921, 12.3, 6.9386) (-10.8096, 12.3, 7.2196) (-10.6139, 12.3, 7.5044) (-10.417, 12.3, 7.7755) (-10.2066, 12.3, 8.0496) (-9.9958, 12.3, 8.31) (-9.7714, 12.3, 8.5727) (-9.5472, 12.3, 8.8217) (-9.3093, 12.3, 9.0724) (-9.0724, 12.3, 9.3093) (-8.8217, 12.3, 9.5472) (-8.5727, 12.3, 9.7714) (-8.31, 12.3, 9.9958) (-8.0496, 12.3, 10.2066) (-7.7755, 12.3, 10.417) (-7.5044, 12.3, 10.6139) (-7.2196, 12.3, 10.8096) (-6.9386, 12.3, 10.9921) (-6.644, 12.3, 11.1727) (-6.3538, 12.3, 11.3402) (-6.0502, 12.3, 11.5051) (-5.7516, 12.3, 11.6572) (-5.4397, 12.3, 11.8059) (-5.1336, 12.3, 11.9422) (-4.8144, 12.3, 12.0745) (-4.5016, 12.3, 12.1945) (-4.1759, 12.3, 12.3099) (-3.8572, 12.3, 12.4134) (-3.5259, 12.3, 12.5116) (-3.2023, 12.3, 12.5983) (-2.8663, 12.3, 12.6789) (-2.5385, 12.3, 12.7486) (-2.1988, 12.3, 12.8116) (-1.8678, 12.3, 12.864) (-1.5253, 12.3, 12.9091) (-1.192, 12.3, 12.9441) (-0.8476, 12.3, 12.9712) (-0.5129, 12.3, 12.9888) (-0.1675, 12.3, 12.9978) (0.1675, 12.3, 12.9978) (0.5129, 12.3, 12.9888) (0.8476, 12.3, 12.9712) (1.192, 12.3, 12.9441) (1.5253, 12.3, 12.9091) (1.8678, 12.3, 12.864) (2.1988, 12.3, 12.8116) (2.5385, 12.3, 12.7486) (2.8663, 12.3, 12.6789) (3.2023, 12.3, 12.5983) (3.5259, 12.3, 12.5116) (3.8572, 12.3, 12.4134) (4.1759, 12.3, 12.3099) (4.5016, 12.3, 12.1945) (4.8144, 12.3, 12.0745) (5.1336, 12.3, 11.9422) (5.4397, 12.3, 11.8059) (5.7516, 12.3, 11.6572) (6.0502, 12.3, 11.5051) (6.3538, 12.3, 11.3402) (6.644, 12.3, 11.1727) (6.9386, 12.3, 10.9921) (7.2196, 12.3, 10.8096) (7.5044, 12.3, 10.6139) (7.7755, 12.3, 10.417) (8.0496, 12.3, 10.2066) (8.31, 12.3, 9.9958) (8.5727, 12.3, 9.7714) (8.8217, 12.3, 9.5472) (9.0724, 12.3, 9.3093) (9.3093, 12.3, 9.0724) (9.5472, 12.3, 8.8217) (9.7714, 12.3, 8.5727) (9.9958, 12.3, 8.31) (10.2066, 12.3, 8.0496) (10.417, 12.3, 7.7755) (10.6139, 12.3, 7.5044) (10.8096, 12.3, 7.2196) (10.9921, 12.3, 6.9386) (11.1727, 12.3, 6.644) (11.3402, 12.3, 6.3538) (11.5051, 12.3, 6.0502) (11.6572, 12.3, 5.7516) (11.8059, 12.3, 5.4397) (11.9422, 12.3, 5.1336) (12.0745, 12.3, 4.8144) (12.1945, 12.3, 4.5016) (12.3099, 12.3, 4.1759) (12.4134, 12.3, 3.8572) (12.5116, 12.3, 3.5259) (12.5983, 12.3, 3.2023) (12.6789, 12.3, 2.8663) (12.7486, 12.3, 2.5385) (12.8116, 12.3, 2.1988) (12.864, 12.3, 1.8678) (12.9091, 12.3, 1.5253) (12.9441, 12.3, 1.192) (12.9712, 12.3, 0.8476) (12.9888, 12.3, 0.5129) (12.9978, 12.3, 0.1675) (12.9978, 12.3, -0.1675) (12.9888, 12.3, -0.5129) (12.9712, 12.3, -0.8476) (12.9441, 12.3, -1.192) (12.9091, 12.3, -1.5253) (12.864, 12.3, -1.8678) (12.8116, 12.3, -2.1988) (12.7486, 12.3, -2.5385) (12.6789, 12.3, -2.8663) (12.5983, 12.3, -3.2023) (12.5116, 12.3, -3.5259) (12.4134, 12.3, -3.8572) (12.3099, 12.3, -4.1759) (12.1945, 12.3, -4.5016) (12.0745, 12.3, -4.8144) (11.9422, 12.3, -5.1336) (11.8059, 12.3, -5.4397) (11.6572, 12.3, -5.7516) (11.5051, 12.3, -6.0502) (11.3402, 12.3, -6.3538) (11.1727, 12.3, -6.644) (10.9921, 12.3, -6.9386) (10.8096, 12.3, -7.2196) (10.6139, 12.3, -7.5044) (10.417, 12.3, -7.7755) (10.2066, 12.3, -8.0496) (9.9958, 12.3, -8.31) (9.7714, 12.3, -8.5727) (9.5472, 12.3, -8.8217) (9.3093, 12.3, -9.0724) (9.0724, 12.3, -9.3093) (8.8217, 12.3, -9.5472) (8.5727, 12.3, -9.7714) (8.31, 12.3, -9.9958) (8.0496, 12.3, -10.2066) (7.7755, 12.3, -10.417) (7.5044, 12.3, -10.6139) (7.2196, 12.3, -10.8096) (6.9386, 12.3, -10.9921) (6.644, 12.3, -11.1727) (6.3538, 12.3, -11.3402) (6.0502, 12.3, -11.5051) (5.7516, 12.3, -11.6572) (5.4397, 12.3, -11.8059) (5.1336, 12.3, -11.9422) (4.8144, 12.3, -12.0745) (4.5016, 12.3, -12.1945) (4.1759, 12.3, -12.3099) (3.8572, 12.3, -12.4134) (3.5259, 12.3, -12.5116) (3.2023, 12.3, -12.5983) (2.8663, 12.3, -12.6789) (2.5385, 12.3, -12.7486) (2.1988, 12.3, -12.8116) (1.8678, 12.3, -12.864) (1.5253, 12.3, -12.9091) (1.192, 12.3, -12.9441) (0.8476, 12.3, -12.9712) (0.5129, 12.3, -12.9888) (0.1675, 12.3, -12.9978) (-0.1675, 12.3, -12.9978) (-0.5129, 12.3, -12.9888) (-0.8476, 12.3, -12.9712) (-1.192, 12.3, -12.9441) (-1.5253, 12.3, -12.9091) (-1.8678, 12.3, -12.864) (-2.1988, 12.3, -12.8116) (-2.5385, 12.3, -12.7486) (-2.8663, 12.3, -12.6789) (-3.2023, 12.3, -12.5983) (-3.5259, 12.3, -12.5116) (-3.8572, 12.3, -12.4134) (-4.1759, 12.3, -12.3099) (-4.5016, 12.3, -12.1945) (-4.8144, 12.3, -12.0745) (-5.1336, 12.3, -11.9422) (-5.4397, 12.3, -11.8059) (-5.7516, 12.3, -11.6572) (-6.0502, 12.3, -11.5051) (-6.3538, 12.3, -11.3402) (-6.644, 12.3, -11.1727) (-6.9386, 12.3, -10.9921) (-7.2196, 12.3, -10.8096) (-7.5044, 12.3, -10.6139) (-7.7755, 12.3, -10.417) (-8.0496, 12.3, -10.2066) (-8.31, 12.3, -9.9958) (-8.5727, 12.3, -9.7714) (-8.8217, 12.3, -9.5472) (-9.0724, 12.3, -9.3093) (-9.3093, 12.3, -9.0724) (-9.5472, 12.3, -8.8217) (-9.7714, 12.3, -8.5727) (-9.9958, 12.3, -8.31) (-10.2066, 12.3, -8.0496) (-10.417, 12.3, -7.7755) (-10.6139, 12.3, -7.5044)
sketch "Sketch4" plane through (0, 12.3, 0) normal (0, 1, 0) x (1, 0, 0)
  circle A0 centre (0, 0) radius 7.5
  dimension "d12" = 15
  constraints: 1 centre point, 1 coincident
  measures "d12" diameter of A0
extrude "Extrusion3" cut sketch "Sketch4" against normal blind 0.8
sketch "Sketch5" plane through (0, 11.5, 0) normal (0, 1, 0) x (1, 0, 0)
  circle A0 centre (-3.5004, 3.4996) radius 1
  circle A1 centre (3.4996, -3.5004) radius 1
  line L0 (-3.5004, 3.4996) -> (3.4996, 3.4996) construction
  line L1 (3.4996, 3.4996) -> (3.4996, -3.5004) construction
  line L2 (3.4996, -3.5004) -> (-3.5004, -3.5004) construction
  line L3 (-3.5004, -3.5004) -> (-3.5004, 3.4996) construction
  point P0 (0, 0)
  dimension "d15" = 2
  dimension "d16" = 2
  dimension "d17" = 7
  dimension "d18" = 7
  constraints: 8 end point, 2 centre point, 2 parallel, 1 horizontal, 1 perpendicular
  measures "d15" diameter of A0
  measures "d16" diameter of A1
  measures "d17" distance of L0.start L0.end
  measures "d18" distance between parallel lines of L2 L0
extrude "Extrusion4" add sketch "Sketch5" along normal blind 2
body "Solid1"
